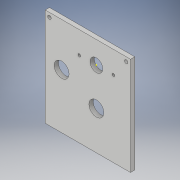
# Autodesk Inventor part: Rack and Pinion Gearbox Plate
Saved by Autodesk Inventor 2018 (Build 220112000, 112)
## iProperties
Created: 2019-01-29
Part Number: Rack and Pinion Gearbox Plate
Material: Generic
Document SubType Name: Modeling
Designer: maste
Density: 1 g/cm^3
Appearance: Default
Author: maste
Autodesk Inventor part; units mm, degrees
ref_plane "YZ Plane" through (0, 0, 0) normal (1, 0, 0) x (0, 1, 0)
ref_plane "XZ Plane" through (0, 0, 0) normal (0, 1, 0) x (-1, 0, 0)
ref_plane "XY Plane" through (0, 0, 0) normal (0, 0, 1) x (1, 0, 0)
sketch "Sketch1" plane through (0, 0, 0) normal (0, 0, 1) x (1, 0, 0)
  circle A0 centre (0, 0) radius 9.525
  line L0 (0, 0) -> (25.4, 0) construction
  line L1 (25.4, 0) -> (-25.4, 0) construction
  line L2 (0, 0) -> (0, -55.88) construction
  line L3 (0, -55.88) -> (-51.7955, -31.7274) construction
  circle A1 centre (0, -55.88) radius 11.1125
  circle A2 centre (-51.7955, -31.7274) radius 11.1125
  line L4 (0, -55.88) -> (0, -106.68) construction
  line L5 (0, -106.68) -> (50.8, -106.68)
  line L6 (50.8, -106.68) -> (50.8, 33.02)
  line L7 (-51.7955, -31.7274) -> (-98.7855, -31.7274) construction
  line L8 (50.8, 33.02) -> (-76.2, 33.02)
  line L9 (-76.2, 33.02) -> (-76.2, -106.68)
  line L10 (-76.2, -106.68) -> (0, -106.68)
  circle A3 centre (25.4, 0) radius 2.0193
  circle A4 centre (-25.4, 0) radius 2.0193
  line L11 (-76.2, 33.02) -> (-69.85, 33.02) construction
  line L12 (-69.85, 33.02) -> (-69.85, 26.67) construction
  circle A5 centre (-69.85, 26.67) radius 2.5797
  line L13 (-12.7, 33.02) -> (-12.7, -106.68) construction
  line L14 (50.8, -36.83) -> (-76.2, -36.83) construction
  circle A6 centre (44.45, 26.67) radius 2.5797
  dimension "d0" = 19.05
  dimension "d1" = 25.4
  dimension "d2" = 50.8
  dimension "d3" = 55.88
  dimension "d4" = 57.15
  dimension "d5" = 65
  dimension "d6" = 22.225
  dimension "d7" = 22.225
  dimension "d8" = 50.8
  dimension "d9" = 50.8
  dimension "d10" = 139.7
  dimension "d11" = 46.99
  dimension "d12" = 127
  dimension "d13" = 4.0386
  dimension "d14" = 6.35
  dimension "d15" = 6.35
  dimension "d16" = 5.1594
  constraints: 30 end point, 7 centre point, 6 coincident, 4 horizontal, 4 perpendicular, 3 midpoint, 3 point on line, 2 vertical, 1 collinear, 1 symmetric about line, 1 other
  measures "d0" diameter of A0
  measures "d1" distance of L0.start L0.end
  measures "d2" distance of L0.end L1.end
  measures "d3" distance of L0.start L2.end
  measures "d4" distance of L2.end L3.end
  measures "d5" angle of L2 L3
  measures "d6" diameter of A1
  measures "d7" diameter of A2
  measures "d8" distance of L4.start L4.end
  measures "d9" distance of L4.end L5.end
  measures "d10" distance of L5.end L6.end
  measures "d11" distance of L7.start L7.end
  measures "d12" distance of L6.end L8.end
  measures "d13" diameter of A3
  measures "d14" distance of L8.end L11.end
  measures "d15" distance of L11.end L12.end
  measures "d16" diameter of A5
extrude "Extrusion1" add sketch "Sketch1" along normal blind 6.35
sketch "Sketch2" plane through (0, 0, 6.35) normal (0, 0, 1) x (1, 0, 0)
  line L0 (-76.2, -106.68) -> (50.8, -106.68) projected
  line L1 (-76.2, -106.68) -> (50.8, -106.68)
  line L2 (50.8, -106.68) -> (50.8, -113.03)
  line L3 (50.8, -113.03) -> (-76.2, -113.03)
  line L4 (-76.2, -113.03) -> (-76.2, -106.68)
  point P0 (0, 0)
  dimension "d19" = 127
  dimension "d20" = 6.35
  constraints: 8 end point, 2 parallel, 1 horizontal, 1 perpendicular
  measures "d19" distance of L2.end L3.end
  measures "d20" distance of L1.end L2.end
extrude "Extrusion2" add sketch "Sketch2" against normal blind 6.35
sketch "Sketch3" plane through (0, 0, 6.35) normal (0, 0, 1) x (1, 0, 0)
  point P0 (0, 0)
body "Solid1"
